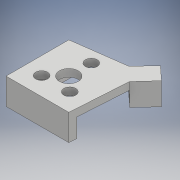
# Autodesk Inventor part: MS_Holderv11
Saved by Autodesk Inventor 2017 (Build 210142000, 142)
## iProperties
Created: 2017-12-14
Part Number: MS_Holderv11
Material: Generic
Document SubType Name: Modeling
Designer: andrew
Density: 1 g/cm^3
Appearance: Default
Author: andrew
Autodesk Inventor part; units mm, degrees
ref_plane "YZ Plane" through (0, 0, 0) normal (1, 0, 0) x (0, 1, 0)
ref_plane "XZ Plane" through (0, 0, 0) normal (0, 1, 0) x (-1, 0, 0)
ref_plane "XY Plane" through (0, 0, 0) normal (0, 0, 1) x (1, 0, 0)
sketch "Sketch1" plane through (0, 0, 0) normal (0, 0, 1) x (1, 0, 0)
  line L0 (3.7674, 2.461) -> (4.3315, 3.068) construction
  line L1 (4.3315, 3.068) -> (2.5, 4.7697) construction
  line L2 (2.5, 4.7697) -> (2.94, 6) construction
  line L3 (2.94, 6) -> (-2, 6) construction
  line L4 (-2, 6) -> (-2, 4.0311) construction
  arc A0 (-2, 4.0311) -> (-3.182, 3.182) centre (0, 0) ccw construction
  line L5 (-3.182, 3.182) -> (-3.182, -3.182) construction
  line L6 (-3.182, -3.182) -> (3.182, -3.182) construction
  arc A1 (3.182, -3.182) -> (3.7674, 2.461) centre (0, 0) ccw construction
  circle A2 centre (0, 0) radius 1.2484
  circle A3 centre (0, 3) radius 0.7934
  circle A4 centre (1.875, -1.75) radius 0.7934
  circle A5 centre (-1.875, -1.75) radius 0.7934
  circle A6 centre (0, 0) radius 4 construction
  line L7 (-2, -4.0311) -> (-2, -3.182) construction
  arc A7 (-2, -4.0311) -> (3.182, -3.182) centre (0, 0) ccw construction
  line L8 (-2, -3.182) -> (3.182, -3.182) construction
  arc A8 (-2, 4.0311) -> (-2, -4.0311) centre (0, 0) ccw construction
  line L9 (-3.182, 3.182) -> (-4.182, 3.182) construction
  line L10 (-4.182, 3.182) -> (-4.182, 4.182) construction
  line L11 (-4.182, 4.182) -> (-3.182, 4.182) construction
  line L12 (-3.182, 4.182) -> (-3.182, 3.182) construction
  line L13 (3.182, -3.182) -> (4.182, -3.182) construction
  line L14 (4.182, -3.182) -> (4.182, -4.182) construction
  line L15 (4.182, -4.182) -> (3.182, -4.182) construction
  line L16 (3.182, -4.182) -> (3.182, -3.182) construction
  line L17 (4.182, -4.182) -> (-4.182, -4.182) construction
  line L18 (-4.182, -4.182) -> (-4.182, -3.182) construction
  line L19 (-4.182, -3.182) -> (4.182, -3.182) construction
  line L20 (4.182, -3.182) -> (4.182, -4.182) construction
  line L21 (-4.182, 4.182) -> (-3.182, 4.182) construction
  line L22 (-3.182, 4.182) -> (-3.182, -4.182) construction
  line L23 (-3.182, -4.182) -> (-4.182, -4.182) construction
  line L24 (-4.182, -4.182) -> (-4.182, 4.182) construction
  line L25 (4.3315, 3.068) -> (6.7138, 5.632) construction
  line L26 (4.3315, 3.068) -> (4.6718, 3.4343) construction
  line L27 (4.6718, 3.4343) -> (2.6832, 5.282) construction
  line L28 (6.7138, 5.632) -> (4.8824, 7.3337) construction
  line L29 (2.5, 4.7697) -> (4.8824, 7.3337) construction
  line L30 (2.8403, 5.136) -> (-3.182, 4.182) construction
  line L31 (4.6718, 3.4343) -> (4.182, -3.182) construction
  circle A9 centre (-3.182, -3.182) radius 0.5 construction
  line L32 (-4.182, 4.182) -> (-4.182, -4.182)
  line L33 (-4.182, -4.182) -> (4.182, -4.182)
  line L34 (4.182, -4.182) -> (4.6718, 3.4343)
  line L35 (6.7138, 5.632) -> (4.6718, 3.4343)
  line L36 (6.7138, 5.632) -> (4.9203, 7.2985)
  line L37 (4.9203, 7.2985) -> (2.8403, 5.136)
  line L38 (2.8403, 5.136) -> (-4.182, 4.182)
  dimension "d0" = 1
  dimension "d1" = 1
  dimension "d2" = 1
  dimension "d3" = 1
  dimension "d4" = 3.5
  dimension "d5" = 0.5
  constraints: 78 end point, 10 centre point, 9 perpendicular, 8 parallel, 8 point on circle, 8 point on line, 4 horizontal, 2 collinear, 1 coincident, 1 tangent
  measures "d0" distance of L10.end L11.end
  measures "d1" distance of L9.end L10.end
  measures "d2" distance of L14.end L15.end
  measures "d3" distance of L13.end L14.end
  measures "d4" distance of L0.end L25.end
  measures "d5" distance of L0.end L26.end
extrude "Extrusion1" add sketch "Sketch1" along normal blind 1
sketch "Sketch2" plane through (0, 0, 1) normal (0, 0, 1) x (1, 0, 0)
  circle A0 centre (0, 0) radius 1.2484
  circle A1 centre (0, 3) radius 0.7934
  line L0 (-3.182, -3.182) -> (3.182, -3.182) construction
  circle A2 centre (0, 0) radius 4 construction
  line L1 (-3.182, 3.182) -> (-3.182, -3.182) construction
  arc A3 (-2, 4.0311) -> (-2, -4.0311) centre (0, 0) ccw construction
  arc A4 (-2, 4.0311) -> (-3.182, 3.182) centre (0, 0) ccw construction
  arc A5 (3.182, -3.182) -> (3.7674, 2.461) centre (0, 0) ccw construction
  line L2 (3.7674, 2.461) -> (4.3315, 3.068) construction
  line L3 (4.3315, 3.068) -> (2.5, 4.7697) construction
  line L4 (-2, -3.182) -> (3.182, -3.182) construction
  arc A6 (-2, -4.0311) -> (3.182, -3.182) centre (0, 0) ccw construction
  line L5 (-2, -4.0311) -> (-2, -3.182) construction
  circle A7 centre (-1.875, -1.75) radius 0.7934
  line L6 (-2, 6) -> (-2, 4.0311) construction
  line L7 (2.5, 4.7697) -> (2.94, 6) construction
  line L8 (2.94, 6) -> (-2, 6) construction
  circle A8 centre (1.875, -1.75) radius 0.7934
  line L9 (-3.182, 3.182) -> (-4.182, 3.182) construction
  line L10 (-4.182, 3.182) -> (-4.182, 4.182) construction
  line L11 (-4.182, 4.182) -> (-3.182, 4.182) construction
  line L12 (-3.182, 4.182) -> (-3.182, 3.182) construction
  line L13 (3.182, -3.182) -> (4.182, -3.182) construction
  line L14 (4.182, -3.182) -> (4.182, -4.182) construction
  line L15 (4.182, -4.182) -> (3.182, -4.182) construction
  line L16 (3.182, -4.182) -> (3.182, -3.182) construction
  line L17 (4.182, -4.182) -> (-4.182, -4.182) construction
  line L18 (-4.182, -4.182) -> (-4.182, -3.182) construction
  line L19 (-4.182, -3.182) -> (4.182, -3.182) construction
  line L20 (4.182, -3.182) -> (4.182, -4.182) construction
  line L21 (-4.182, 4.182) -> (-3.182, 4.182) construction
  line L22 (-3.182, 4.182) -> (-3.182, -4.182) construction
  line L23 (-3.182, -4.182) -> (-4.182, -4.182) construction
  line L24 (-4.182, -4.182) -> (-4.182, 4.182) construction
  line L25 (4.3315, 3.068) -> (6.7138, 5.632) construction
  line L26 (4.3315, 3.068) -> (4.6718, 3.4343) construction
  line L27 (4.6718, 3.4343) -> (2.6832, 5.282) construction
  line L28 (6.7138, 5.632) -> (4.8824, 7.3337) construction
  line L29 (2.5, 4.7697) -> (4.8824, 7.3337) construction
  line L30 (2.8403, 5.136) -> (-3.182, 4.182) construction
  line L31 (4.6718, 3.4343) -> (4.182, -3.182) construction
  arc A9 (-3.182, -2.682) -> (-2.682, -3.182) centre (-3.182, -3.182) ccw
  line L32 (-4.182, 4.182) -> (-4.182, -4.182)
  line L33 (-4.182, -4.182) -> (4.182, -4.182)
  line L34 (4.182, -4.182) -> (4.6718, 3.4343)
  line L35 (6.7138, 5.632) -> (4.6718, 3.4343)
  line L36 (6.7138, 5.632) -> (4.9203, 7.2985)
  line L37 (4.9203, 7.2985) -> (2.8403, 5.136)
  line L38 (2.8403, 5.136) -> (-4.182, 4.182)
  line L39 (-3.182, -2.682) -> (-3.182, 4.3178)
  line L40 (2.8403, 5.136) -> (-4.182, 4.182) projected
  line L41 (-2.682, -3.182) -> (4.2463, -3.182)
  dimension "d8" = 1
  dimension "d9" = 1
  dimension "d10" = 1
  dimension "d11" = 1
  dimension "d12" = 3.5
  dimension "d13" = 0.5
  constraints: 82 end point, 13 point on line, 10 centre point, 10 perpendicular, 10 point on circle, 8 parallel, 4 horizontal, 2 collinear, 1 coincident, 1 tangent, 1 vertical
  measures "d8" distance of L10.end L11.end
  measures "d9" distance of L9.end L10.end
  measures "d10" distance of L14.end L15.end
  measures "d11" distance of L13.end L14.end
  measures "d12" distance of L2.end L25.end
  measures "d13" distance of L2.end L26.end
extrude "Extrusion2" add sketch "Sketch2" along normal blind 2.5 contours A9 L41 L34 L33 L32 L38 L39
sketch "Sketch3" plane through (0, 0, 1) normal (0, 0, 1) x (1, 0, 0)
  circle A0 centre (0, 0) radius 1.2484
  circle A1 centre (0, 3) radius 0.7934
  line L0 (-3.182, -3.182) -> (3.182, -3.182) construction
  circle A2 centre (0, 0) radius 4 construction
  line L1 (-3.182, 3.182) -> (-3.182, -3.182) construction
  arc A3 (-2, 4.0311) -> (-2, -4.0311) centre (0, 0) ccw construction
  arc A4 (-2, 4.0311) -> (-3.182, 3.182) centre (0, 0) ccw construction
  arc A5 (3.182, -3.182) -> (3.7674, 2.461) centre (0, 0) ccw construction
  line L2 (3.7674, 2.461) -> (4.3315, 3.068) construction
  line L3 (4.3315, 3.068) -> (2.5, 4.7697) construction
  line L4 (-2, -3.182) -> (3.182, -3.182) construction
  arc A6 (-2, -4.0311) -> (3.182, -3.182) centre (0, 0) ccw construction
  line L5 (-2, -4.0311) -> (-2, -3.182) construction
  circle A7 centre (-1.875, -1.75) radius 0.7934
  line L6 (-2, 6) -> (-2, 4.0311) construction
  line L7 (2.5, 4.7697) -> (2.94, 6) construction
  line L8 (2.94, 6) -> (-2, 6) construction
  circle A8 centre (1.875, -1.75) radius 0.7934
  line L9 (-3.182, 3.182) -> (-4.182, 3.182) construction
  line L10 (-4.182, 3.182) -> (-4.182, 4.182) construction
  line L11 (-4.182, 4.182) -> (-3.182, 4.182) construction
  line L12 (-3.182, 4.182) -> (-3.182, 3.182) construction
  line L13 (3.182, -3.182) -> (4.182, -3.182) construction
  line L14 (4.182, -3.182) -> (4.182, -4.182) construction
  line L15 (4.182, -4.182) -> (3.182, -4.182) construction
  line L16 (3.182, -4.182) -> (3.182, -3.182) construction
  line L17 (4.182, -4.182) -> (-4.182, -4.182) construction
  line L18 (-4.182, -4.182) -> (-4.182, -3.182) construction
  line L19 (-4.182, -3.182) -> (4.182, -3.182) construction
  line L20 (4.182, -3.182) -> (4.182, -4.182) construction
  line L21 (-4.182, 4.182) -> (-3.182, 4.182) construction
  line L22 (-3.182, 4.182) -> (-3.182, -4.182) construction
  line L23 (-3.182, -4.182) -> (-4.182, -4.182) construction
  line L24 (-4.182, -4.182) -> (-4.182, 4.182) construction
  line L25 (4.3315, 3.068) -> (6.7138, 5.632) construction
  line L26 (4.3315, 3.068) -> (4.6718, 3.4343) construction
  line L27 (4.6718, 3.4343) -> (2.6832, 5.282) construction
  line L28 (6.7138, 5.632) -> (4.8824, 7.3337) construction
  line L29 (2.5, 4.7697) -> (4.8824, 7.3337) construction
  line L30 (2.8403, 5.136) -> (-3.182, 4.182) construction
  line L31 (4.6718, 3.4343) -> (4.182, -3.182) construction
  circle A9 centre (-3.182, -3.182) radius 0.5 construction
  line L32 (-4.182, 4.182) -> (-4.182, -4.182)
  line L33 (-4.182, -4.182) -> (4.182, -4.182)
  line L34 (4.182, -4.182) -> (4.6718, 3.4343)
  line L35 (6.7138, 5.632) -> (4.6718, 3.4343)
  line L36 (6.7138, 5.632) -> (4.9203, 7.2985)
  line L37 (4.9203, 7.2985) -> (2.8403, 5.136)
  line L38 (2.8403, 5.136) -> (-4.182, 4.182)
  line L39 (2.8403, 5.136) -> (-3.182, 4.3178) projected
  line L40 (4.2463, -3.182) -> (4.6718, 3.4343) projected
  line L41 (2.8403, 5.136) -> (4.6718, 3.4343)
  dimension "d16" = 1
  dimension "d17" = 1
  dimension "d18" = 1
  dimension "d19" = 1
  dimension "d20" = 3.5
  dimension "d21" = 0.5
  constraints: 80 end point, 10 centre point, 9 perpendicular, 8 parallel, 8 point on circle, 8 point on line, 4 horizontal, 2 collinear, 1 coincident, 1 tangent
  measures "d16" distance of L10.end L11.end
  measures "d17" distance of L9.end L10.end
  measures "d18" distance of L14.end L15.end
  measures "d19" distance of L13.end L14.end
  measures "d20" distance of L2.end L25.end
  measures "d21" distance of L2.end L26.end
extrude "Extrusion3" add sketch "Sketch3" along normal blind 2 contours L37 L36 L35 L41
sketch "Sketch4" plane through (4.9203, 7.2985, 3) normal (0.6807, 0.7326, 0) x (0.7326, -0.6807, 0)
  line L0 (2.4482, 2) -> (-0.0518, 2) construction
  line L1 (2.4482, 2) -> (2.4482, 0) construction
  line L2 (-0.0518, 0) -> (2.4482, 0) construction
  line L3 (-0.0518, 2) -> (-0.0518, 0) construction
  line L4 (2.4482, 0) -> (0, 0) construction
  line L5 (1.2241, 0) -> (-0.0518, 0) construction
  line L6 (-0.0518, 0) -> (-0.0518, 1) construction
  line L7 (-0.0518, 1) -> (1.2241, 1) construction
  line L8 (1.2241, 1) -> (1.2241, 0) construction
  circle A0 centre (1.2241, 1) radius 0.65
  dimension "d24" = 1.3
  constraints: 8 end point, 2 midpoint, 2 parallel, 1 centre point, 1 coincident, 1 horizontal, 1 perpendicular
  measures "d24" diameter of A0
extrude "Extrusion4" cut sketch "Sketch4" against normal blind 3
sketch "Sketch5" plane through (0, 0, 0) normal (0, 0, -1) x (-1, 0, 0)
  line L0 (4.182, 4.182) -> (4.182, -4.182) projected
  line L1 (4.182, -4.182) -> (-4.182, -4.182) projected
  line L2 (-4.182, -4.182) -> (-4.2463, -3.182) projected
  line L3 (-4.2463, -3.182) -> (2.682, -3.182) projected
  arc A0 (2.682, -3.182) -> (3.182, -2.682) centre (3.182, -3.182) ccw projected
  line L4 (3.182, -2.682) -> (3.182, 4.3178) projected
  line L5 (3.182, 4.3178) -> (4.182, 4.182) projected
  point P0 (0, 0)
extrude "Extrusion5" add sketch "Sketch5" along normal blind 2.5
sketch "Sketch6" plane through (0, 0, 0) normal (0, 0, -1) x (-1, 0, 0)
  line L0 (-6.7138, 5.632) -> (-4.9203, 7.2985) projected
  line L1 (-4.9203, 7.2985) -> (-2.8403, 5.136) projected
  line L2 (-2.8403, 5.136) -> (-4.6718, 3.4343) projected
  line L3 (-4.6718, 3.4343) -> (-6.7138, 5.632) projected
  point P0 (0, 0)
extrude "Extrusion6" add sketch "Sketch6" along normal blind 2
sketch "Sketch7" plane through (4.9203, 7.2985, 3) normal (0.6807, 0.7326, 0) x (0.7326, -0.6807, 0)
  line L0 (2.4482, 5) -> (-0.0518, 5) projected
  circle A0 centre (1.2241, 4) radius 0.65
  point P0 (1.3634, 3)
  constraints: 1 centre point
extrude "Extrusion7" cut sketch "Sketch7" against normal blind 4
sketch "Sketch8" plane through (0, 0, 3.5) normal (0, 0, 1) x (1, 0, 0)
  line L0 (-4.9294, -4.4454) -> (7.7152, -4.4454)
  line L1 (7.7152, -4.4454) -> (7.7152, 7.9918)
  line L2 (7.7152, 7.9918) -> (-4.9294, 7.9918)
  line L3 (-4.9294, 7.9918) -> (-4.9294, -4.4454)
  point P0 (0, 0)
  constraints: 8 end point, 2 parallel, 1 horizontal, 1 perpendicular
extrude "Extrusion8" cut sketch "Sketch8" against normal blind 2.5
body "Solid1"
